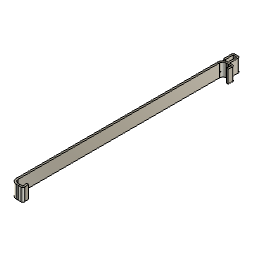
hook (Autodesk Fusion 360 design; units mm, degrees)
Autodesk Fusion 360 part; units mm, degrees
note: some values were not read from the file. Chosen so that the rebuilt part matches the saved one: which bodies a step acts on; which face or edge a step refers to. Set by a fixed rule: which sketch regions a step uses.
sketch "Sketch1" plane through (0, 0, 0) normal (0, 0, 1) x (1, 0, 0)
  line L0 (4, 0) -> (9.2, 0)
  line L1 (9.2, -5.0191) -> (9.2, -237.9809)
  line L2 (9.2, -243) -> (4, -243)
  line L3 (0, -239) -> (0, -4)
  line L4 (6, 2) -> (9.2, 2)
  line L5 (9.2, -245) -> (4, -245)
  line L6 (-2, -239) -> (-2, -4)
  line L7 (9.2, 0) -> (9.2, 2)
  arc A0 (0, -239) -> (4, -243) centre (4, -239) ccw
  arc A1 (4, 0) -> (0, -4) centre (4, -4) ccw
  arc A2 (4, 2) -> (-2, -4) centre (4, -4) ccw
  arc A3 (-2, -239) -> (4, -245) centre (4, -239) ccw
  line L8 (9.2, 0) -> (8.7642, -4.981)
  line L9 (9.2, 0) -> (14.2, 0) construction
  line L10 (11.1924, -0.1743) -> (10.7566, -5.1553)
  line L11 (8.7642, -4.981) -> (10.7566, -5.1553)
  line L12 (9.2, 0) -> (11.2, 0)
  arc A4 (11.1924, -0.1743) -> (9.2, 2) centre (9.2, 0) ccw
  line L13 (9.2, -243) -> (8.7642, -238.019)
  line L14 (8.7642, -238.019) -> (10.7566, -237.8447)
  line L15 (11.1924, -242.8257) -> (10.7566, -237.8447)
  arc A5 (9.2, -245) -> (11.1924, -242.8257) centre (9.2, -243) ccw
  line L16 (9.2, -243) -> (9.2, -243)
  line L17 (-2, 12) -> (-2, 4)
  line L18 (0, 4) -> (0, 12)
  line L19 (0, 12) -> (4, 12)
  line L20 (-0.0003, 14) -> (4.0004, 14)
  line L21 (6, 12) -> (6, 2)
  line L22 (4, 12) -> (4, 2)
  line L23 (0, 4) -> (0, 2)
  line L24 (0, 2) -> (-2, 2)
  line L25 (-2, 2) -> (-2, 4)
  arc A6 (0.0003, 14) -> (-2, 12) centre (0, 12) ccw
  arc A7 (6, 12) -> (3.9996, 14) centre (4, 12) ccw
  point P0 (0, -243)
  dimension "d1" = 9.2
  dimension "d2" = 243
  dimension "d4" = 4
  dimension "d5" = 6
  dimension "d6" = 95
  dimension "d7" = 5
  dimension "d8" = -2
  dimension "d9" = 2
  dimension "d13" = 2
  dimension "d14" = 8
  dimension "d16" = 4
  dimension "d18" = 2
  dimension "d19" = 2
  constraint horizontal L0
  constraint vertical L1
  constraint horizontal L2
  constraint vertical L3
  constraint perpendicular L4 L7
  constraint coincident P0 L2
  constraint coincident P0 L3
  constraint tangent L2 A0
  constraint tangent L3 A0
  constraint coincident origin L0
  constraint coincident origin L3
  constraint tangent L0 A1
  constraint tangent L3 A1
  constraint equal A0 A1
  constraint tangent L4 A2
  constraint tangent L6 A2
  constraint tangent L5 A3
  constraint tangent L6 A3
  constraint equal A2 A3
  constraint horizontal L9
  constraint perpendicular L10 L11
  constraint perpendicular L1 L12
  constraint coincident L0.end L7.start
  constraint coincident L12.end A4
  constraint coincident L11 L1.start
  constraint coincident L2.start L13.start
  constraint coincident L14 L1.end
  constraint perpendicular L18 L19
  constraint perpendicular L17 L20
  constraint perpendicular L4 L21
  constraint vertical L23
  constraint horizontal L24
  constraint vertical L25
  constraint coincident L18.end L19.start
  constraint tangent L17 A6
  constraint coincident L19.end L22.start
  constraint tangent L21 A7
  constraint coincident L20.start A6
  constraint coincident L20 A6.start
  constraint coincident L20 A7.end
  constraint coincident A7 L20.end
  measures "d1" distance of origin L0.end
  measures "d2" distance of origin P0
  measures "d4" radius of A0
  measures "d5" radius of A2
  measures "d6" angle of L8 L9
  measures "d7" distance of L0.end L8.end
  measures "d9" distance of L0.end L12.end
  measures "d13" distance of L17.end L18.start
  measures "d14" distance of L18.start L18.end
  measures "d16" distance of L18.end L19.end
  measures "d18" distance of L17.end L18.start
  measures "d19" distance of L17.end L24.end
extrude "Extrude1" add sketch "Sketch1" along normal blind 15 contours L0 L2 L3 L4 L5 L6 L7 A0 A1 A2 A3 L13 L14 L15 A5 L17 L18 L19 L20 L21 L22 L23 L24 L25 A6 A7 makes body 1
extrude "Extrude2" add sketch "Sketch1" along normal blind 15 contours L8 L10 L11 L12 A4 | L7 L12 A4 bodies 1
split "Split1" by plane through (6, 12, 0) normal (1, 0, 0) bodies 1 makes body 2 at (9.0547, -1.6603, 5) makes body 3 at (9.0547, -241.3397, 5)
move_body "Move1" bodies 2 3 to x (1, 0, 0) y (0, 1, 0) z (0, 0, 1) at (0.4, 0, 0)
extrude "Extrude3" add 2 faces at (6.4, 1.3333, 5) (6.4, -244.3333, 5) along direction (-1, 0, 0) blind 1 on bodies 2 3 bodies 1 2 3
sketch "Sketch2" plane through (-2, 0, 0) normal (-1, 0, 0) x (0, -1, 0)
  line L0 (-12, 0) -> (-2, 0)
  line L1 (-2, 0) -> (-2, 15)
  line L2 (-2, 15) -> (-12, 15)
  line L3 (-12, 15) -> (-12, 0)
  line L4 (-2, 7.5) -> (-6, 7.5)
  line L5 (-6, 7.5) -> (-2, 3.5)
  line L6 (-6, 7.5) -> (-0.3431, 7.5) construction
  line L7 (-6, 7.5) -> (-2, 11.5)
  line L8 (-2, 7.5) -> (-2, 9.25)
  line L9 (-2, 9.25) -> (-12, 9.25)
  line L10 (-12, 9.25) -> (-12, 5.75)
  line L11 (-12, 5.75) -> (-2, 5.75)
  line L12 (-2, 5.75) -> (-2, 9.25)
  line L13 (-8.0282, 9.25) -> (-8.0282, 5.75)
  dimension "d26" = 4
  dimension "d27" = 45
  dimension "d28" = 90
  dimension "d29" = 1.75
  dimension "d30" = 3.5
  constraint midpoint L1 L4.start
  constraint perpendicular L1 L4
  constraint horizontal L6
  constraint coincident L1 L5.end
  constraint coincident L1 L7.end
  constraint perpendicular L6 L8
  constraint horizontal L9
  constraint vertical L10
  constraint horizontal L11
  constraint vertical L12
  constraint coincident L9 L13.start
  constraint coincident L11 L13.end
  constraint perpendicular L11 L13
  measures "d26" distance of L4.start L4.end
  measures "d27" angle of L5 L6
  measures "d28" angle of L5 L7
  measures "d29" distance of L4.start L8.end
  measures "d30" distance of L8.end L11.end
extrude "Extrude4" cut sketch "Sketch2" against normal blind 2 contours L1 L5 L11 | L5 L7 L9 L11 L13 | L1 L4 L5 L11 L12 | L1 L4 L7 L8 L9 L12 | L1 L7 L9 bodies 1
extrude "Extrude5" cut 1 faces at (-1.3333, 8.0282, 8.0833) along direction (0, 1, 0) blind 1 on bodies 1 bodies 1
split "Split2" by plane through (-2, 9.0282, 9.25) normal (0, -1, 0) bodies 1 makes body 4 at (0, -160.6667, 5) makes body 5 at (0, 7.4355, 11.1667) makes body 6 at (0, 7.4355, 3.8333)
move_body "Move2" bodies 6 5 to x (1, 0, 0) y (0, 1, 0) z (0, 0, 1) at (0, 1, 0)
combine "Combine1" operation add target body 4 tool bodies 5 6 1
box "BoxPrimitive1" add length 12.9765 width 2 height -0.5 placed x (0, 1, 0) y (-1, 0, 0) z (0, 0, 1) at (0, -3.9483, 5.75) separate body makes body 7
